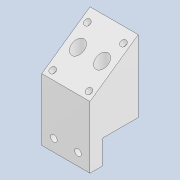
# Autodesk Inventor part: s_base1
Saved by Autodesk Inventor 2022 (Build 260153000, 153)
## iProperties
Created: 2021-08-20
Part Number: s_base1
Material: ABS プラスチック
Document SubType Name: Modeling
Designer: yuta0
Density: 1.06 g/cm^3
Appearance: 滑らか - 白
Mass: 90.1717 g
Surface Area: 175.133 cm^2
Volume: 85.0677 cm^3
Author: yuta0
Autodesk Inventor part; units mm, degrees
ref_plane "YZ Plane" through (0, 0, 0) normal (1, 0, 0) x (0, 1, 0)
ref_plane "XZ Plane" through (0, 0, 0) normal (0, 1, 0) x (-1, 0, 0)
sketch "スケッチ1" plane through (0, 0, 0) normal (1, 0, 0) x (0, 1, 0)
  line L0 (0, 0) -> (51.545, 0)
  line L1 (51.545, 0) -> (79.5533, -40)
  line L2 (79.5533, -40) -> (0, -40)
  line L3 (0, -40) -> (0, 0)
  line L4 (0, -10) -> (20, -10)
  line L5 (20, -10) -> (20, -40)
  line L6 (20, -40) -> (0, -40)
  line L7 (0, -40) -> (0, -10)
  point P0 (0, -40)
  dimension "d0" = 35
  dimension "d1" = 51.545
  dimension "d2" = 40
  dimension "d53" = 10
  dimension "d54" = 0
  dimension "d55" = 20
  constraints: 16 end point, 3 parallel, 2 horizontal, 2 perpendicular, 1 point on line
  measures "d0" angle of L3 L1
  measures "d1" distance of L0.start L0.end
  measures "d2" distance of L2.end L0.start
  measures "d53" distance between parallel lines of L0 L4
  measures "d54" distance between parallel lines of L2 L6
  measures "d55" distance of L4.start L4.end
extrude "押し出し1" add sketch "スケッチ1" along normal mid plane 40 contours L0 L1 L2 L5 L4 L3
ref_plane "作業平面1" through (-20, 70, -40) normal (0, -1, 0) x (1, 0, 0)
sketch "スケッチ3" plane through (-20, 70, -40) normal (0, -1, 0) x (1, 0, 0)
  line L0 (0, 0) -> (40, 0) projected
  line L1 (0, 40) -> (0, 0) projected
  line L2 (40, 0) -> (40, 40) projected
  point P0 (20, 40)
  point P1 (10, 20)
  point P2 (30, 20)
  dimension "d12" = 10
  dimension "d13" = 10
  dimension "d73" = 20
  constraints: 1 horizontal alignment
  measures "d12" distance from line of L1 point (10, 20)
  measures "d13" distance from line of L2 point (30, 20)
  measures "d73" distance from line of L0 point (10, 20)
hole "穴1" at (-10, 70, -20) at (10, 70, -20) direction (0, -1, 0) diameter 5.5 end through all counterbore diameter 10 counterbore depth 15 clearance for "Socket Head Cap Screw" size "M5" standard "Ansi Metric M Profile"
sketch "スケッチ4" plane through (-20, 51.545, 0) normal (0, 0.819152, 0.5735764) x (1, 0, 0)
  line L0 (35, 5) -> (5, 5)
  line L1 (5, 5) -> (5, 40)
  line L2 (5, 40) -> (35, 40)
  line L3 (35, 40) -> (35, 5)
  line L4 (0, 48.831) -> (40, 48.831) projected
  line L5 (40, 0) -> (0, 0) projected
  line L6 (0, 0) -> (0, 48.831) projected
  line L7 (40, 48.831) -> (40, 0) projected
  point P0 (20, -29.565)
  dimension "d22" = 48.831
  dimension "d36" = 5
  dimension "d46" = 5
  dimension "d51" = 40
  dimension "d52" = 5
  dimension "d57" = 35
  constraints: 8 end point, 2 parallel, 1 horizontal, 1 perpendicular
  measures "d22" distance of L5.start L4.end
  measures "d36" distance between parallel lines of L5 L0
  measures "d46" distance between parallel lines of L6 L1
  measures "d51" distance of L4.start L4.end
  measures "d52" distance between parallel lines of L7 L3
  measures "d57" distance of L2.end L0.start
hole "穴2" at (15, 74.4881, -32.7661) at (15, 54.4129, -4.0958) at (-15, 74.4881, -32.7661) at (-15, 54.4129, -4.0958) direction (0, -0.819152, -0.5735764) diameter 5 depth 6 tip angle 118
fillet "フィレット3" radius 1 1 edges at (0, 20, -10)
sketch "スケッチ7" plane through (-20, 51.545, 0) normal (0, 0, 1) x (1, 0, 0)
  line L0 (0, -51.545) -> (0, 0) projected
  line L1 (40, 0) -> (40, -51.545) projected
  line L2 (0, -51.545) -> (40, -51.545) projected
  point P0 (20, -51.545)
  point P1 (10, -41.545)
  point P2 (30, -41.545)
  point P3 (0, -50.545)
  point P4 (40, -50.545)
  dimension "d63" = 10
  dimension "d64" = 10
  dimension "d76" = 10
  dimension "d77" = 10
  measures "d63" distance from line of L0 point (10, -41.545)
  measures "d64" distance from line of L1 point (30, -41.545)
  measures "d76" distance from line of L2 point (10, -41.545)
  measures "d77" distance from line of L2 point (30, -41.545)
hole "穴3" at (-10, 10, 0) at (10, 10, 0) direction (0, 0, -1) diameter 5.5 end through all clearance for "Socket Head Cap Screw" size "M5" standard "Ansi Metric M Profile"
sketch "スケッチ8" plane through (20, 79.5533, -40) normal (0, 0, -1) x (-1, 0, 0)
  line L0 (40, -59.5533) -> (0, -59.5533) projected
  point P0 (20, -79.5533)
  point P1 (20, -51.5533)
  point P2 (20, -10.5533)
  dimension "d78" = 41
  dimension "d79" = 8
  constraints: 1 vertical alignment
  measures "d78" distance of point (20, -51.553) point (20, -10.553)
  measures "d79" distance from line of L0 point (20, -51.553)
hole "穴4" at (0, 28, -40) at (0, 69, -40) direction (0, 0, 1) diameter 5 depth 6 tip angle 118
equation "\"d13\" = d12"
equation "\"d63\" = d62"
equation "\"d64\" = d63"
equation "\"d62\" = 10"
